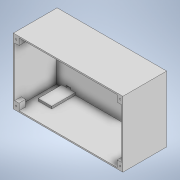
# Autodesk Inventor part: Box
Saved by Autodesk Inventor 2022 (Build 260153000, 153)
## iProperties
Created: 2021-07-04
Part Number: Box
Material: Generic
Document SubType Name: Modeling
Designer: Matthijs
Density: 1 g/cm^3
Appearance: Default
Author: Matthijs
Autodesk Inventor part; units mm, degrees
ref_plane "YZ Plane" through (0, 0, 0) normal (1, 0, 0) x (0, 1, 0)
ref_plane "XZ Plane" through (0, 0, 0) normal (0, 1, 0) x (-1, 0, 0)
ref_plane "XY Plane" through (0, 0, 0) normal (0, 0, 1) x (1, 0, 0)
sketch "Sketch7" plane through (0, 0, 0) normal (0, 0, 1) x (1, 0, 0)
  line L0 (125, -75) -> (-125, -75)
  line L1 (-125, -75) -> (-125, 75)
  line L2 (-125, 75) -> (125, 75)
  line L3 (125, 75) -> (125, -75)
  line L4 (125, -75) -> (-125, 75) construction
  line L5 (-125, -75) -> (125, 75) construction
  point P0 (0, 0)
  dimension "d15" = 250
  dimension "d16" = 150
  constraints: 12 end point, 2 midpoint, 2 parallel, 1 horizontal, 1 perpendicular
  measures "d15" distance of L1.end L2.end
  measures "d16" distance of L0.end L1.end
extrude "Box Outside" add sketch "Sketch7" along normal blind 100
sketch "Sketch8" plane through (0, 0, 100) normal (0, 0, 1) x (1, 0, 0)
  line L0 (-122, 72) -> (122, 72)
  line L1 (122, 72) -> (122, -72)
  line L2 (122, -72) -> (-122, -72)
  line L3 (-122, -72) -> (-122, 72)
  line L4 (125, 75) -> (-125, 75) projected
  line L5 (-125, 75) -> (-125, -75) projected
  line L6 (-125, -75) -> (125, -75) projected
  line L7 (125, -75) -> (125, 75) projected
  point P0 (0, 0)
  dimension "d19" = 3
  dimension "d20" = 3
  dimension "d21" = 3
  dimension "d22" = 3
  constraints: 8 end point, 2 parallel, 1 horizontal, 1 perpendicular
  measures "d19" distance between parallel lines of L4 L0
  measures "d20" distance between parallel lines of L5 L3
  measures "d21" distance between parallel lines of L6 L2
  measures "d22" distance between parallel lines of L7 L1
extrude "Box Cut" cut sketch "Sketch8" against normal blind 95 contours L0 L1 L2 L3
sketch "Sketch9" plane through (-122, -72, 100) normal (0, 1, 0) x (1, 0, 0)
  line L0 (0, 0) -> (10, 0)
  line L1 (10, 0) -> (10, 15)
  line L2 (10, 15) -> (0, 15)
  line L3 (0, 15) -> (0, 0)
  point P0 (122, 100)
  dimension "d25" = 10
  dimension "d26" = 15
  constraints: 8 end point, 2 parallel, 1 horizontal, 1 perpendicular
  measures "d25" distance of L2.end L1.end
  measures "d26" distance of L1.end L0.end
extrude "ScrewHole Box LB" add sketch "Sketch9" along normal blind 15
sketch "Sketch10" plane through (-122, -72, 5) normal (0, 1, 0) x (1, 0, 0)
  line L0 (244, -95) -> (244, 0) projected
  line L1 (244, -95) -> (234, -95)
  line L2 (234, -95) -> (234, -80)
  line L3 (234, -80) -> (244, -80)
  line L4 (244, -80) -> (244, -95)
  point P0 (122, 5)
  dimension "d29" = 10
  dimension "d30" = 15
  constraints: 8 end point, 2 parallel, 1 horizontal, 1 perpendicular
  measures "d29" distance of L2.end L3.end
  measures "d30" distance of L1.end L2.end
extrude "ScrewHole Box RB" add sketch "Sketch10" along normal blind 15
sketch "Sketch11" plane through (-122, 72, 100) normal (0, -1, 0) x (1, 0, 0)
  line L0 (0, 0) -> (244, 0) projected
  line L1 (0, 0) -> (10, 0)
  line L2 (10, 0) -> (10, -15)
  line L3 (10, -15) -> (0, -15)
  line L4 (0, -15) -> (0, 0)
  point P0 (122, -100)
  dimension "d33" = 10
  dimension "d34" = 15
  constraints: 8 end point, 2 parallel, 1 horizontal, 1 perpendicular
  measures "d33" distance of L2.end L3.end
  measures "d34" distance of L1.end L2.end
extrude "ScrewHole Box LU" add sketch "Sketch11" along normal blind 15
sketch "Sketch13" plane through (122, -72, 5) normal (-1, 0, 0) x (0, 0, 1)
  line L0 (95, 144) -> (0, 144) projected
  line L1 (95, 144) -> (80, 144)
  line L2 (80, 144) -> (80, 129)
  line L3 (80, 129) -> (95, 129)
  line L4 (95, 129) -> (95, 144)
  point P0 (-5, 72)
  dimension "d37" = 15
  dimension "d38" = 15
  constraints: 8 end point, 2 parallel, 1 horizontal, 1 perpendicular
  measures "d37" distance of L3.end L2.end
  measures "d38" distance of L2.end L1.end
extrude "ScrewHole Box RU" add sketch "Sketch13" along normal blind 10
sketch "Sketch27" plane through (0, 0, 100) normal (0, 0, 1) x (1, 0, 0)
  line L0 (-112, -72) -> (-112, -57) projected
  line L1 (-125, 75) -> (-125, -75) projected
  line L2 (-112, -57) -> (-125, -57)
  line L3 (-125, -57) -> (-125, -75)
  line L4 (-125, -75) -> (-112, -75)
  line L5 (-112, -75) -> (-112, -57)
  line L6 (-112, -57) -> (-125, -75)
  line L7 (-112, -75) -> (-125, -57)
  circle A0 centre (-118.5, -66) radius 2.4
  point P0 (0, 0)
  dimension "d84" = 4.8
  constraints: 12 end point, 2 parallel, 1 centre point, 1 coincident, 1 horizontal, 1 midpoint, 1 perpendicular
  measures "d84" diameter of A0
extrude "Outside ScrewHole LB" cut sketch "Sketch27" against normal blind 26 contours A0 L7 L6 | L6 L7 A0 | A0 L6 L7 | L7 L6 A0
sketch "Sketch29" plane through (0, 0, 100) normal (0, 0, 1) x (1, 0, 0)
  line L0 (-112, -72) -> (-112, -57) projected
  line L1 (-125, -75) -> (125, -75) projected
  line L2 (-112, -57) -> (-125, -57)
  line L3 (-125, -57) -> (-125, -75)
  line L4 (-125, -75) -> (-112, -75)
  line L5 (-112, -75) -> (-112, -57)
  line L6 (-112, -57) -> (-125, -75)
  circle A0 centre (-118.5, -66) radius 2.4
  point P0 (0, 0)
  constraints: 10 end point, 2 parallel, 1 centre point, 1 coincident, 1 horizontal, 1 midpoint, 1 perpendicular
extrude "ScrewRibbon LB" add sketch "Sketch29" against normal blind 2 contours A0 L6 | L6 A0
sketch "Sketch30" plane through (0, 0, 100) normal (0, 0, 1) x (1, 0, 0)
  line L0 (-122, -57) -> (-112, -57) projected
  line L1 (-125, -75) -> (125, -75) projected
  line L2 (-112, -57) -> (-125, -57)
  line L3 (-125, -57) -> (-125, -75)
  line L4 (-125, -75) -> (-112, -75)
  line L5 (-112, -75) -> (-112, -57)
  line L6 (-112, -57) -> (-125, -75)
  circle A0 centre (-118.5, -66) radius 1.7
  point P0 (0, 0)
  dimension "d92" = 3.4
  constraints: 10 end point, 2 parallel, 1 centre point, 1 coincident, 1 horizontal, 1 midpoint, 1 perpendicular
  measures "d92" diameter of A0
extrude "Inside ScrewHole LB" cut sketch "Sketch30" against normal blind 24 contours A0 L6 | L6 A0
sketch "Sketch31" plane through (0, 0, 100) normal (0, 0, 1) x (1, 0, 0)
  line L0 (-125, 75) -> (-125, -75) projected
  line L1 (-112, 57) -> (-122, 57) projected
  line L2 (-125, 75) -> (-112, 75)
  line L3 (-112, 75) -> (-112, 57)
  line L4 (-112, 57) -> (-125, 57)
  line L5 (-125, 57) -> (-125, 75)
  line L6 (-125, 75) -> (-112, 57)
  circle A0 centre (-118.5, 66) radius 2.4
  point P0 (0, 0)
  dimension "d95" = 4.8
  constraints: 10 end point, 2 parallel, 1 centre point, 1 coincident, 1 horizontal, 1 midpoint, 1 perpendicular
  measures "d95" diameter of A0
extrude "Outside ScrewHole LU" cut sketch "Sketch31" against normal blind 24 contours A0 L6 | L6 A0
sketch "Sketch32" plane through (0, 0, 100) normal (0, 0, 1) x (1, 0, 0)
  line L0 (-122, 57) -> (-112, 57) projected
  line L1 (-125, 75) -> (-125, -75) projected
  line L2 (-112, 57) -> (-125, 57)
  line L3 (-125, 57) -> (-125, 75)
  line L4 (-125, 75) -> (-112, 75)
  line L5 (-112, 75) -> (-112, 57)
  line L6 (-112, 75) -> (-125, 57)
  circle A0 centre (-118.5, 66) radius 2.4
  point P0 (0, 0)
  dimension "d98" = 4.8
  constraints: 10 end point, 2 parallel, 1 centre point, 1 coincident, 1 horizontal, 1 midpoint, 1 perpendicular
  measures "d98" diameter of A0
extrude "ScrewRibbon LU" add sketch "Sketch32" against normal blind 2 contours A0 L6 | L6 A0
sketch "Sketch33" plane through (0, 0, 100) normal (0, 0, 1) x (1, 0, 0)
  line L0 (125, 75) -> (-125, 75) projected
  line L1 (-112, 57) -> (-122, 57) projected
  line L2 (-125, 75) -> (-112, 75)
  line L3 (-112, 75) -> (-112, 57)
  line L4 (-112, 57) -> (-125, 57)
  line L5 (-125, 57) -> (-125, 75)
  line L6 (-125, 75) -> (-112, 57)
  circle A0 centre (-118.5, 66) radius 1.7
  point P0 (0, 0)
  dimension "d101" = 3.4
  constraints: 10 end point, 2 parallel, 1 centre point, 1 coincident, 1 horizontal, 1 midpoint, 1 perpendicular
  measures "d101" diameter of A0
extrude "Inside ScrewHole LU" cut sketch "Sketch33" against normal blind 21.75 contours A0 L6 | L6 A0
sketch "Sketch34" plane through (0, 0, 100) normal (0, 0, 1) x (1, 0, 0)
  line L0 (112, 57) -> (112, 72) projected
  line L1 (125, 75) -> (-125, 75) projected
  line L2 (112, 57) -> (125, 57)
  line L3 (125, 57) -> (125, 75)
  line L4 (125, 75) -> (112, 75)
  line L5 (112, 75) -> (112, 57)
  line L6 (125, 75) -> (112, 57)
  circle A0 centre (118.5, 66) radius 2.4
  point P0 (0, 0)
  dimension "d104" = 4.8
  constraints: 10 end point, 2 parallel, 1 centre point, 1 coincident, 1 horizontal, 1 midpoint, 1 perpendicular
  measures "d104" diameter of A0
extrude "Outside ScrewHole RU" cut sketch "Sketch34" against normal blind 21.75 contours A0 L6 | L6 A0
sketch "Sketch35" plane through (0, 0, 100) normal (0, 0, 1) x (1, 0, 0)
  line L0 (125, -75) -> (125, 75) projected
  line L1 (122, 57) -> (112, 57) projected
  line L2 (125, 75) -> (112, 75)
  line L3 (112, 75) -> (112, 57)
  line L4 (112, 57) -> (125, 57)
  line L5 (125, 57) -> (125, 75)
  line L6 (125, 75) -> (-125, 75) projected
  line L7 (125, 75) -> (112, 57)
  circle A0 centre (118.5, 66) radius 2.4
  point P0 (0, 0)
  dimension "d107" = 4.8
  constraints: 10 end point, 2 parallel, 1 centre point, 1 coincident, 1 horizontal, 1 midpoint, 1 perpendicular
  measures "d107" diameter of A0
extrude "ScrewRibbon RU" add sketch "Sketch35" against normal blind 2 contours A0 L7 | L7 A0
sketch "Sketch36" plane through (0, 0, 100) normal (0, 0, 1) x (1, 0, 0)
  line L0 (122, 57) -> (112, 57) projected
  line L1 (125, -75) -> (125, 75) projected
  line L2 (112, 57) -> (125, 57)
  line L3 (125, 57) -> (125, 75)
  line L4 (125, 75) -> (112, 75)
  line L5 (112, 75) -> (112, 57)
  line L6 (112, 57) -> (125, 75)
  circle A0 centre (118.5, 66) radius 2.4 projected
  circle A1 centre (118.5, 66) radius 1.7
  point P0 (0, 0)
  dimension "d110" = 3.4
  constraints: 10 end point, 2 coincident, 2 parallel, 1 centre point, 1 horizontal, 1 perpendicular
  measures "d110" diameter of A1
extrude "Inside ScrewHole RU" cut sketch "Sketch36" against normal blind 20 contours A1 L6 | L6 A1
sketch "Sketch37" plane through (0, 0, 100) normal (0, 0, 1) x (1, 0, 0)
  line L0 (125, -75) -> (125, 75) projected
  line L1 (112, -72) -> (112, -57) projected
  line L2 (125, -75) -> (112, -75)
  line L3 (112, -75) -> (112, -57)
  line L4 (112, -57) -> (125, -57)
  line L5 (125, -57) -> (125, -75)
  line L6 (112, -75) -> (125, -57)
  circle A0 centre (118.5, -66) radius 2.4
  point P0 (0, 0)
  dimension "d113" = 4.8
  constraints: 10 end point, 2 parallel, 1 centre point, 1 coincident, 1 horizontal, 1 midpoint, 1 perpendicular
  measures "d113" diameter of A0
extrude "Outside ScrewHole RB" cut sketch "Sketch37" against normal blind 20 contours A0 L6 | L6 A0
sketch "Sketch38" plane through (0, 0, 100) normal (0, 0, 1) x (1, 0, 0)
  line L0 (122, -57) -> (112, -57) projected
  line L1 (125, -75) -> (125, 75) projected
  line L2 (112, -57) -> (125, -57)
  line L3 (125, -57) -> (125, -75)
  line L4 (125, -75) -> (112, -75)
  line L5 (112, -75) -> (112, -57)
  line L6 (125, -57) -> (112, -75)
  circle A0 centre (118.5, -66) radius 2.4
  point P0 (0, 0)
  dimension "d116" = 4.8
  constraints: 10 end point, 2 parallel, 1 centre point, 1 coincident, 1 horizontal, 1 midpoint, 1 perpendicular
  measures "d116" diameter of A0
extrude "ScrewRibbon RB" add sketch "Sketch38" against normal blind 2 contours A0 L6 | L6 A0
sketch "Sketch39" plane through (0, 0, 100) normal (0, 0, 1) x (1, 0, 0)
  line L0 (112, -72) -> (112, -57) projected
  line L1 (125, -75) -> (125, 75) projected
  line L2 (112, -57) -> (125, -57)
  line L3 (125, -57) -> (125, -75)
  line L4 (125, -75) -> (112, -75)
  line L5 (112, -75) -> (112, -57)
  line L6 (112, -75) -> (125, -57)
  circle A0 centre (118.5, -66) radius 2.4 projected
  circle A1 centre (118.5, -66) radius 1.7
  point P0 (0, 0)
  dimension "d119" = 3.4
  constraints: 10 end point, 2 coincident, 2 parallel, 1 centre point, 1 horizontal, 1 perpendicular
  measures "d119" diameter of A1
extrude "Inside ScrewHole RB" cut sketch "Sketch39" against normal blind 20 contours A1 L6 | L6 A1
sketch "Sketch42" plane through (-122, -72, 5) normal (0, 1, 0) x (1, 0, 0)
  line L0 (244, 0) -> (0, 0) projected
  line L1 (12.5963, 0) -> (43.5963, 0)
  line L2 (43.5963, 0) -> (43.5963, -54)
  line L3 (43.5963, -54) -> (12.5963, -54)
  line L4 (12.5963, -54) -> (12.5963, 0)
  point P0 (122, 5)
  point P1 (43.5963, 0)
  dimension "d134" = 31
  dimension "d135" = 54
  constraints: 8 end point, 2 parallel, 1 horizontal, 1 perpendicular, 1 point on line
  measures "d134" distance of L2.end L3.end
  measures "d135" distance of L1.end L2.end
extrude "ESPHolder" add sketch "Sketch42" along normal blind 5
sketch "Sketch43" plane through (0, 0, 5) normal (0, 0, 1) x (1, 0, 0)
  line L0 (-109.4037, -67) -> (-78.4037, -67) projected
  line L1 (-99.1037, -67) -> (-88.7037, -67)
  line L2 (-88.7037, -67) -> (-88.7037, -62.5)
  line L3 (-88.7037, -62.5) -> (-99.1037, -62.5)
  line L4 (-99.1037, -62.5) -> (-99.1037, -67)
  line L5 (-78.4037, -67) -> (-109.4037, -67)
  line L6 (-109.4037, -67) -> (-109.4037, -51.7804)
  line L7 (-109.4037, -51.7804) -> (-78.4037, -51.7804)
  line L8 (-78.4037, -51.7804) -> (-78.4037, -67)
  point P0 (0, 0)
  dimension "d138" = 10.3
  dimension "d139" = 10.3
  dimension "d140" = 4.5
  constraints: 16 end point, 4 parallel, 2 horizontal, 2 perpendicular, 1 point on line
  measures "d138" distance between parallel lines of L8 L2
  measures "d139" distance between parallel lines of L6 L4
  measures "d140" distance between parallel lines of L0 L3
extrude "PortHole" cut sketch "Sketch43" against normal through all contours L4 L3 L2 L0
body "Solid2"
